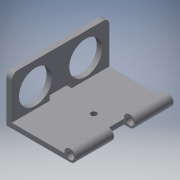
# Autodesk Inventor part: Lid, Explosion Button
Saved by Autodesk Inventor 2016 (Build 200138000, 138)
## iProperties
Created: 2016-03-16
Part Number: Lid, Explosion Button
Material: Generic
Document SubType Name: Modeling
Designer: Owner
Density: 1 g/cm^3
Appearance: Default
Author: Owner
Autodesk Inventor part; units mm, degrees
ref_plane "YZ Plane" through (0, 0, 0) normal (1, 0, 0) x (0, 1, 0)
ref_plane "XZ Plane" through (0, 0, 0) normal (0, 1, 0) x (-1, 0, 0)
ref_plane "XY Plane" through (0, 0, 0) normal (0, 0, 1) x (1, 0, 0)
sketch "Sketch1" plane through (0, 0, 0) normal (0, 0, 1) x (1, 0, 0)
  line L0 (0, 0) -> (3.81, 0)
  line L1 (0, 0) -> (0, 1.27)
  arc A0 (3.81, 0) -> (1.359061, 1.27) centre (3.81, 3) ccw
  circle A1 centre (3.81, 3) radius 1.9
  line L2 (0, 1.27) -> (1.359061, 1.27)
  dimension "d0" = 3.81
  dimension "d1" = 1.27
  dimension "d2" = 6
  dimension "d3" = 3.8
  constraints: 6 end point, 2 centre point, 2 point on circle, 1 coincident, 1 horizontal, 1 perpendicular, 1 tangent, 1 vertical
  measures "d0" distance of L0.start L0.end
  measures "d1" distance of L0.start L1.end
  measures "d2" diameter of A0
  measures "d3" diameter of A1
extrude "Extrusion1" add sketch "Sketch1" along normal blind 30.48
ref_plane "Work Plane1" through (0, 0, 20.32) normal (0, 0, 1) x (1, 0, 0)
sketch "Sketch2" plane through (0, 0, 20.32) normal (0, 0, 1) x (1, 0, 0)
  arc A0 (3.81, 0) -> (1.359061, 1.27) centre (3.81, 3) ccw
  line L0 (2.54, 1.27) -> (2.54, 0)
  line L1 (0, 0) -> (3.81, 0)
  line L2 (2.54, 0) -> (3.81, 0)
  circle A1 centre (3.81, 3) radius 0.762
  constraints: 4 end point, 1 centre point, 1 coincident, 1 horizontal, 1 point on line, 1 tangent, 1 vertical, 1 other
sketch "Sketch2 outline for Extrusion2" plane through (0, 0, 20.32) normal (0, 0, 1) x (1, 0, 0)
  line L0 (2.54, 0) -> (3.81, 0)
  line L1 (1.359061, 1.27) -> (2.54, 0)
  arc A0 (3.81, 0) -> (1.359061, 1.27) centre (3.81, 3) ccw
  circle A1 centre (3.81, 3) radius 0.762
extrude "Extrusion2" cut sketch "Sketch2 outline for Extrusion2" against normal blind 10.16
sketch "Sketch3" plane through (0, 1.27, 0) normal (0, 1, 0) x (1, 0, 0)
  line L0 (0, 0) -> (3.81, 0)
  line L1 (0, 0) -> (2.531995, 0)
  line L2 (2.531995, 0) -> (-25.408005, 0)
  line L3 (-25.408005, 0) -> (-25.408005, -27.94)
  line L4 (-25.408005, -27.94) -> (2.531995, -27.94)
  line L5 (1.359061, 0) -> (1.359061, -10.16)
  line L6 (1.359061, 0) -> (1.359061, -1.27)
  line L7 (1.359061, -1.27) -> (-25.310939, -1.27)
  line L8 (1.359061, -20.32) -> (1.359061, -30.48)
  line L9 (1.359061, -30.48) -> (1.359061, -29.21)
  line L10 (1.359061, -29.21) -> (-25.310939, -29.21)
  line L11 (-25.310939, -29.21) -> (-25.310939, -1.27)
  line L12 (0.085059, -1.27) -> (0.085059, -29.21)
  line L13 (0, 0) -> (0, -30.48)
  line L14 (0, -1.27) -> (0, -29.21)
  line L15 (1.359061, -29.21) -> (1.359061, -30.48)
  line L16 (1.359061, 0) -> (1.359061, -1.27)
  line L17 (1.359061, -30.48) -> (1.359061, -29.21)
  line L18 (1.359061, -30.48) -> (6.81, -30.48)
  line L19 (1.359061, -30.48) -> (-1.399798, -27.94)
  line L20 (1.359061, -30.48) -> (1.359061, -29.21)
  line L21 (1.359061, -29.21) -> (-1.466488, -29.21)
  point P0 (3.81, -30.48)
  dimension "d9" = 27.94
  dimension "d10" = 27.94
  dimension "d11" = 27.94
  dimension "d12" = 1.27
  dimension "d13" = 26.67
  dimension "d14" = 1.27
  dimension "d15" = 26.67
  constraints: 34 end point, 12 point on line, 5 perpendicular, 4 collinear
  measures "d9" distance of L1.end L2.end
  measures "d10" distance of L2.end L3.end
  measures "d11" distance of L3.end L4.end
  measures "d12" distance of L5.start L6.end
  measures "d13" distance of L6.end L7.end
  measures "d14" distance of L8.end L9.end
  measures "d15" distance of L9.end L10.end
extrude "Extrusion3" cut sketch "Sketch3" against normal blind 25.4 contours L7 L12 L4 L13 | L4 L12 L10 L13
sketch "Sketch4" plane through (0, 0, 0) normal (0, -1, 0) x (1, 0, 0)
  line L0 (1.359061, 0) -> (1.359061, 10.16)
  line L1 (1.359061, 0) -> (-29.120939, 0)
  line L2 (-29.120939, 0) -> (-29.120939, 30.48)
  line L3 (-29.120939, 30.48) -> (1.359061, 30.48)
  line L4 (1.359061, 30.48) -> (1.359061, 0)
  line L5 (0, 1.27) -> (0.085059, 1.27)
  line L6 (0.085059, 1.27) -> (-27.854941, 1.27)
  line L7 (-27.854941, 1.27) -> (-27.854941, 29.21)
  line L8 (-27.854941, 29.21) -> (0.085059, 29.21)
  line L9 (0.085059, 29.21) -> (0.085059, 1.27)
  point P0 (0, 0)
  dimension "d18" = 30.48
  dimension "d19" = 30.48
  dimension "d20" = 30.48
  dimension "d21" = 27.94
  dimension "d22" = 27.94
  dimension "d23" = 27.94
  constraints: 16 end point, 3 perpendicular, 2 horizontal, 1 vertical
  measures "d18" distance of L0.start L1.end
  measures "d19" distance of L1.end L2.end
  measures "d20" distance of L2.end L3.end
  measures "d21" distance of L5.end L6.end
  measures "d22" distance of L6.end L7.end
  measures "d23" distance of L7.end L8.end
sketch "Sketch5" plane through (0, 1.27, 0) normal (0, 1, 0) x (1, 0, 0)
  line L0 (1.359061, 0) -> (0, 0)
  line L1 (1.359061, 0) -> (0, 0)
  line L2 (0, 0) -> (0, -1.27)
  line L3 (0, 0) -> (0, -1.27)
  line L4 (0, -1.27) -> (1.359061, -1.27)
  line L5 (1.359061, 0) -> (1.359061, -10.16)
  line L6 (0, -29.21) -> (0, -30.48)
  line L7 (0, -29.21) -> (2.54, -29.21)
  line L8 (2.54, -29.21) -> (2.54, -30.48)
  line L9 (2.54, -30.48) -> (0, -30.48)
  line L10 (0, -30.48) -> (0, -29.21)
  constraints: 14 end point, 5 perpendicular, 1 collinear, 1 horizontal, 1 point on line
extrude "Extrusion4" cut sketch "Sketch5" against normal blind 25.4
sketch "Sketch6" plane through (1.359061, 1.27, 20.32) normal (0, 1, 0) x (1, 0, 0)
  line L0 (0, 19.05) -> (0, 10.16)
  line L1 (0, 0) -> (0, 10.16)
  line L2 (0, 19.05) -> (0, -8.89)
  line L3 (-1.274003, -8.89) -> (-1.274003, 19.05)
  line L4 (0, -8.89) -> (-1.274003, -8.89)
  line L5 (-1.274003, -8.89) -> (-1.274003, 19.05)
  line L6 (-1.274003, 19.05) -> (0, 19.05)
  point P0 (-1.359061, 20.32)
  constraints: 8 end point, 3 perpendicular, 1 vertical
extrude "Extrusion5" cut sketch "Sketch6" against normal blind 25.4
extrude "Extrusion6" add sketch "Sketch4" against normal blind 1.27
sketch "Sketch7" plane through (0, 1.27, 0) normal (0, 1, 0) x (1, 0, 0)
  line L0 (1.359061, -29.21) -> (1.359061, -30.48)
  line L1 (-29.120939, 0) -> (-29.120939, -30.48)
  line L2 (2.54, 0) -> (-29.120939, 0)
  line L3 (-29.120939, 0) -> (-29.120939, -30.48)
  line L4 (-29.120939, -30.48) -> (2.54, -30.48)
  line L5 (2.54, -30.48) -> (2.54, 0)
  point P0 (0, 0)
  point P1 (2.54, -9.31335)
  constraints: 8 end point, 2 parallel, 1 horizontal, 1 perpendicular, 1 other
extrude "Extrusion7" add sketch "Sketch7" along normal blind 1.27
sketch "Sketch8" plane through (0, 2.54, 0) normal (0, 1, 0) x (1, 0, 0)
  line L0 (-22.120939, 7.26) -> (-22.120939, -37.74)
  line L1 (-29.120939, 0) -> (-29.120939, -30.48)
  line L2 (-29.120939, 0) -> (-29.120939, -30.48)
  line L3 (-29.120939, 0) -> (-26.370939, 0)
  line L4 (-26.370939, 0) -> (-26.370939, -30.48)
  line L5 (-26.370939, -30.48) -> (-29.120939, -30.48)
  line L6 (-29.120939, -30.48) -> (-29.120939, 0)
  point P0 (0, 0)
  dimension "d32" = 2.75
  constraints: 8 end point, 2 parallel, 1 horizontal, 1 perpendicular
  measures "d32" distance of L1.start L3.end
extrude "Extrusion8" add sketch "Sketch8" along normal blind 22
sketch "Sketch9" plane through (0, 0, 0) normal (0, 0, -1) x (-1, 0, 0)
  arc A0 (-0.845476, 2.54) -> (-3.81, 0) centre (-3.81, 3) ccw
  line L0 (29.120939, 0) -> (-3.81, 0)
  line L1 (29.120939, 0) -> (29.120939, 24.54)
  line L2 (26.370939, 24.54) -> (29.120939, 24.54)
  line L3 (26.370939, 2.54) -> (26.370939, 24.54)
  line L4 (-0.845476, 2.54) -> (26.370939, 2.54)
  line L5 (-2.54, 1.586812) -> (-2.54, 2.54)
  arc A1 (-1.966525, 2.54) -> (-2.54, 1.586812) centre (-3.81, 3) ccw
  line L6 (-2.54, 2.54) -> (-1.966525, 2.54)
  point P0 (0, 0)
extrude "Extrusion9" add sketch "Sketch9" along normal blind 10
sketch "Sketch10" plane through (0, 0, 30.48) normal (0, 0, 1) x (1, 0, 0)
  line L0 (0.085059, 1.27) -> (-27.854941, 1.27)
  line L1 (-26.370939, 2.54) -> (2.54, 2.54)
  line L2 (2.54, 0) -> (3.81, 0)
  arc A0 (3.81, 0) -> (0.845476, 2.54) centre (3.81, 3) ccw
  line L3 (2.54, 1.586812) -> (2.54, 2.54)
  line L4 (1.966525, 2.54) -> (2.54, 2.54)
  line L5 (-26.370939, 2.54) -> (-26.370939, 24.54)
  line L6 (-29.120939, 24.54) -> (-26.370939, 24.54)
  line L7 (-29.120939, 0) -> (-29.120939, 24.54)
  arc A1 (2.54, 1.586812) -> (1.966525, 2.54) centre (3.81, 3) ccw
  line L8 (1.359061, 1.27) -> (2.54, 1.27)
  line L9 (2.54, 1.27) -> (2.54, 0)
  line L10 (-26.370939, 2.54) -> (0.845476, 2.54)
  line L11 (-29.120939, 0) -> (1.359061, 0)
  line L12 (1.359061, 0) -> (1.359061, 1.27)
  point P0 (0, 0)
extrude "Extrusion10" add sketch "Sketch10" along normal blind 10
fillet "Fillet1" radius 3.175 2 edges at (-27.7459, 24.54, -10) (-27.7459, 24.54, 40.48)
sketch "Sketch12" plane through (0, 0, 40.48) normal (0, 0, 1) x (1, 0, 0)
  line L0 (2.54, 1.27) -> (2.54, 0)
  line L1 (1.359061, 1.27) -> (2.54, 1.27)
  line L2 (1.359061, 1.27) -> (1.359061, 0)
  line L3 (2.54, 0) -> (1.359061, 0)
  line L4 (2.54, 1.27) -> (2.54, 0)
  line L5 (2.54, 1.27) -> (1.359061, 1.27)
  point P0 (0, 0)
extrude "Extrusion12" add sketch "Sketch12" against normal blind 12
sketch "Sketch13" plane through (0, 0, 40.48) normal (0, 0, 1) x (1, 0, 0)
  arc A0 (2.54, 1.586812) -> (1.966525, 2.54) centre (3.81, 3) ccw
  circle A1 centre (3.81, 3) radius 2
  point P0 (0, 0)
  constraints: 1 centre point, 1 coincident
extrude "Extrusion13" cut sketch "Sketch13" against normal blind 5054.6
sketch "Sketch14" plane through (0, 0, 20.32) normal (0, 0, -1) x (-1, 0, 0)
  arc A0 (-1.863619, 2.54) -> (-2.54, 1.454976) centre (-3.81, 3) ccw
  line L0 (-1.863619, 2.54) -> (-0.845476, 2.54)
  arc A1 (-0.845476, 2.54) -> (-3.81, 0) centre (-3.81, 3) ccw
  line L1 (-2.54, 0) -> (-3.81, 0)
  line L2 (-1.359061, 1.27) -> (-2.54, 0)
  line L3 (-1.359061, 1.27) -> (-2.54, 1.27)
  line L4 (-2.54, 1.27) -> (-2.54, 1.454976)
  line L5 (-2.54, 1.27) -> (-2.54, 0)
  line L6 (-2.54, 1.27) -> (-1.359061, 1.27)
  line L7 (-0.845476, 2.54) -> (26.370939, 2.54)
  line L8 (-1.359061, 1.27) -> (-2.54, 0)
  point P0 (0, 0)
  constraints: 6 end point, 1 parallel
extrude "Extrusion14" add sketch "Sketch14" along normal blind 15 contours L3 L2 L5
sketch "Sketch15" plane through (0, 2.54, 0) normal (0, 1, 0) x (1, 0, 0)
  line L0 (0.845476, 10) -> (0.845476, -10.16)
  line L1 (1.81, -40.48) -> (1.81, 10)
  line L2 (0.845476, -10.16) -> (1.81, -10.16)
  line L3 (1.81, -10.16) -> (1.81, -20.32)
  line L4 (1.81, -20.32) -> (0.845476, -20.32)
  line L5 (0.845476, -20.32) -> (0.845476, -10.16)
  line L6 (0.845476, -10.16) -> (12.384081, -10.16)
  line L7 (12.384081, -10.16) -> (12.384081, -20.32)
  line L8 (12.384081, -20.32) -> (0.845476, -20.32)
  line L9 (0.845476, -20.32) -> (0.845476, -10.16)
  point P0 (0, 0)
  constraints: 16 end point, 4 parallel, 2 horizontal, 2 perpendicular, 1 point on line
extrude "Extrusion15" cut sketch "Sketch15" against normal blind 15
sketch "Sketch16" plane through (-29.120939, 0, -10) normal (-1, 0, 0) x (0, 0, 1)
  circle A0 centre (12.24, 12.54) radius 8 projected
  circle A1 centre (38.24, 12.54) radius 8 projected
  circle A2 centre (12.24, 12.54) radius 8.5
  circle A3 centre (38.24, 12.54) radius 8.5
  point P0 (10, 0)
  dimension "d54" = 17
  dimension "d55" = 17
  constraints: 2 centre point, 2 coincident
  measures "d54" diameter of A2
  measures "d55" diameter of A3
extrude "Extrusion16" cut sketch "Sketch16" against normal blind 25.4 contours A0 | A1 | A2 | A3
sketch "Sketch17" plane through (0, 0, 10.16) normal (0, 0, 1) x (1, 0, 0)
  line L0 (3.81, 0) -> (0.845476, 0)
  arc A0 (3.81, 0) -> (0.845476, 2.54) centre (3.81, 3) ccw
  line L1 (0.845476, 2.54) -> (0.845476, 0)
  circle A1 centre (3.81, 3) radius 2
  point P0 (0, 0)
extrude "Extrusion17" cut sketch "Sketch17" against normal blind 0.5
sketch "Sketch18" plane through (0, 0, 20.32) normal (0, 0, -1) x (-1, 0, 0)
  circle A0 centre (-3.81, 3) radius 2
  line L0 (-0.845476, 0) -> (-3.81, 0)
  line L1 (-0.845476, 2.54) -> (-0.845476, 0)
  arc A1 (-0.845476, 2.54) -> (-3.81, 0) centre (-3.81, 3) ccw
  point P0 (0, 0)
extrude "Extrusion18" cut sketch "Sketch18" against normal blind 0.5
sketch "Sketch19" plane through (-29.120939, 0, -10) normal (0, -1, 0) x (1, 0, 0)
  line L0 (29.205997, 11.27) -> (1.265997, 11.27)
  line L1 (1.265997, 11.27) -> (1.265997, 39.21)
  line L2 (1.265997, 39.21) -> (29.205997, 39.21)
  line L3 (29.205997, 39.21) -> (29.205997, 11.27)
  point P0 (29.120939, 10)
  constraints: 8 end point, 2 parallel, 1 horizontal, 1 perpendicular
extrude "Extrusion19" add sketch "Sketch19" against normal blind 2.032
sketch "Sketch20" plane through (-29.120939, 0, -10) normal (-1, 0, 0) x (0, 0, 1)
  line L0 (0, 2.54) -> (50.48, 2.54) projected
  line L1 (25.24, 2.54) -> (30.828, 2.54)
  line L2 (30.828, 2.54) -> (19.652, 2.54)
  line L3 (19.652, 2.54) -> (30.828, 2.54)
  line L4 (30.828, 2.54) -> (30.828, 5.08)
  line L5 (30.828, 5.08) -> (19.652, 5.08)
  line L6 (19.652, 5.08) -> (19.652, 2.54)
  point P0 (10, 0)
  dimension "d64" = 5.588
  dimension "d65" = 11.176
  dimension "d66" = 2.54
  constraints: 12 end point, 2 parallel, 2 point on line, 1 horizontal, 1 midpoint, 1 perpendicular
  measures "d64" distance of L1.start L1.end
  measures "d65" distance of L1.end L2.end
  measures "d66" distance of L3.end L4.end
extrude "Extrusion20" cut sketch "Sketch20" against normal blind 25.4
fillet "Fillet2" radius 0.25 4 edges at (-27.7459, 5.08, 9.652) (-27.7459, 2.54, 9.652) (-27.7459, 2.54, 20.828) (-27.7459, 5.08, 20.828)
sketch "Sketch21" plane through (0, 2.54, 0) normal (0, 1, 0) x (1, 0, 0)
  line L0 (0.845476, -9.66) -> (0.845476, -20.82)
  line L1 (0.845476, -15.24) -> (-4.154524, -15.24)
  line L2 (-4.154524, -15.24) -> (-9.154524, -15.24)
  circle A0 centre (-9.154524, -15.24) radius 1.5
  point P0 (0, 0)
  dimension "d70" = 5
  dimension "d71" = 5
  dimension "d72" = 3
  constraints: 4 end point, 1 centre point, 1 coincident, 1 horizontal, 1 midpoint, 1 point on line
  measures "d70" distance of L1.start L1.end
  measures "d71" distance of L1.end L2.end
  measures "d72" diameter of A0
extrude "Extrusion21" cut sketch "Sketch21" against normal blind 25.4
body "Solid1"
